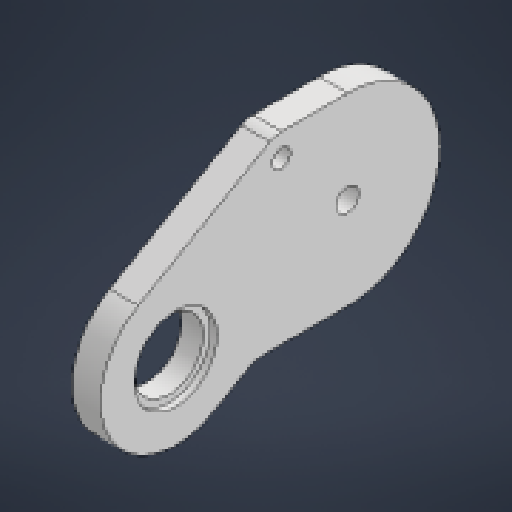
# Autodesk Inventor part: GearCover
Saved by Autodesk Inventor 2024.2 (Build 282272000, 272)
## iProperties
Created: 2023-12-29
Part Number: GearCover
Material: 一般
Document SubType Name: モデリング
Designer: Hanaoka
Density: 1 g/cm^3
Appearance: 既定
Sheet Metal Rule: Default
Author: Hanaoka
Autodesk Inventor part; units mm, degrees
ref_plane "YZ Plane" through (0, 0, 0) normal (1, 0, 0) x (0, 1, 0)
ref_plane "XZ Plane" through (0, 0, 0) normal (0, 1, 0) x (-1, 0, 0)
ref_plane "XY Plane" through (0, 0, 0) normal (0, 0, 1) x (1, 0, 0)
sketch "スケッチ1" plane through (0, 0, 0) normal (1, 0, 0) x (0, 1, 0)
  circle A0 centre (-4.4971, 14.9328) radius 3.6
  circle A1 centre (-4.4971, 14.9328) radius 3
  arc A2 (1.1321, 18.1828) -> (-10.1263, 11.6828) centre (-4.4971, 14.9328) ccw
  line L0 (-10.1263, 11.6828) -> (-8.4019, 8.6962)
  line L1 (-8, 7.1962) -> (-8, 0)
  line L2 (8, 0) -> (8, 5.7513)
  line L3 (7.7321, 6.7513) -> (1.1321, 18.1828)
  circle A3 centre (-4.4971, 14.9328) radius 5 construction
  arc A4 (8, 5.7513) -> (7.7321, 6.7513) centre (6, 5.7513) ccw
  circle A5 centre (6, 5.7513) radius 0.8
  circle A6 centre (6, 5.7513) radius 2 construction
  arc A7 (-8, 0) -> (8, 0) centre (0, 0) ccw
  circle A8 centre (0, 0) radius 1
  line L4 (-8, 8) -> (-8, 0) construction
  line L5 (-8, 0) -> (0, 0) construction
  circle A9 centre (0, 0) radius 2.5 construction
  line L6 (0, -14.3624) -> (0, 30.1744) projected
  line L7 (-4.4971, 14.9328) -> (0, 0) construction
  arc A10 (-8, 7.1962) -> (-8.4019, 8.6962) centre (-11, 7.1962) ccw
  circle A11 centre (2.5, -4.3301) radius 1.25
  line L8 (2.5, -4.3301) -> (0, 0) construction
  point P0 (8, 6.2872)
  dimension "d0" = 6
  dimension "d1" = 7.2
  dimension "d2" = 6.5
  dimension "d7" = 10
  dimension "d9" = 2
  dimension "d10" = 1.6
  dimension "d11" = 4
  dimension "d13" = 150
  dimension "d14" = 8
  dimension "d15" = 2
  dimension "d18" = 13.2
  dimension "d19" = 8
  dimension "d20" = 8
  dimension "d21" = 5
  dimension "d26" = 3
  dimension "d27" = 2.5
  dimension "d28" = 30
  dimension "d29" = 5
  constraints: 16 end point, 12 centre point, 8 coincident, 8 point on circle, 8 tangent, 4 point on line, 2 parallel, 1 perpendicular, 1 vertical
  measures "d0" diameter of A1
  measures "d1" diameter of A0
  measures "d2" radius of A2
  measures "d7" diameter of A3
  measures "d9" radius of A4
  measures "d10" diameter of A5
  measures "d11" diameter of A6
  measures "d13" angle of L1 L0
  measures "d14" radius of A7
  measures "d15" diameter of A8
  measures "d18" distance of L3.start L3.end
  measures "d19" distance of L4.end L5.end
  measures "d20" distance of L4.start L4.end
  measures "d21" diameter of A9
  measures "d26" radius of A10
  measures "d27" diameter of A11
  measures "d28" angle of L6 L8
  measures "d29" distance of L8.start L7.end
extrude "押し出し3" add sketch "スケッチ1" along normal blind 2.5 contours A0 | L3 A4 L2 A7 L6 A8 A2 | L6 A8 A7 L1 A10 L0 A2 | A11
sketch "スケッチ2" plane through (2.5, 0, 0) normal (1, 0, 0) x (0, 0, -1)
  line L0 (0, 8) -> (-5.7513, 8) projected
  arc A0 (-5.7513, 8) -> (-6.7513, 7.7321) centre (-5.7513, 6) ccw projected
  line L1 (-6.7513, 7.7321) -> (-18.1828, 1.1321) projected
  arc A1 (-18.1828, 1.1321) -> (-11.6828, -10.1263) centre (-14.9328, -4.4971) ccw projected
  line L2 (-11.6828, -10.1263) -> (-8.6962, -8.4019) projected
  arc A2 (-7.1962, -8) -> (-8.6962, -8.4019) centre (-7.1962, -11) ccw projected
  line L3 (-7.1962, -8) -> (0, -8) projected
  arc A3 (0, -8) -> (0, 8) centre (0, 0) ccw projected
  circle A4 centre (0, 0) radius 1 projected
  circle A5 centre (-5.7513, 6) radius 0.8 projected
  circle A6 centre (-14.9328, -4.4971) radius 3 projected
  circle A7 centre (-14.9328, -4.4971) radius 3.6
  dimension "d32" = 7.2
  constraints: 1 centre point, 1 coincident
  measures "d32" diameter of A7
extrude "押し出し4" cut sketch "スケッチ2" against normal blind 0.6 contours A7
